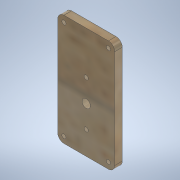
# Autodesk Inventor part: 上下直動t5.5_エンコーダ軸受け_CPY
Saved by Autodesk Inventor 2020.3 (Build 243373000, 373)
## iProperties
Created: 2020-07-07
Part Number: 上下直動t5.5_エンコーダ軸受け_CPY
Material: 木材 (カエデ材)
Document SubType Name: Modeling
Designer: totot
Density: 0.67 g/cm^3
Appearance: ナチュラル カエデ材 - 光沢 濃い着色
Author: totot
Autodesk Inventor part; units mm, degrees
ref_plane "YZ Plane" through (0, 0, 0) normal (1, 0, 0) x (0, 1, 0)
ref_plane "XZ Plane" through (0, 0, 0) normal (0, 1, 0) x (-1, 0, 0)
ref_plane "XY Plane" through (0, 0, 0) normal (0, 0, 1) x (1, 0, 0)
sketch "スケッチ1" plane through (0, 0, 0) normal (0, 0, 1) x (1, 0, 0)
  line L0 (0, 0) -> (41, 0)
  line L1 (41, 0) -> (41, -80)
  line L2 (41, -80) -> (0, -80)
  line L3 (0, -80) -> (0, 0)
  dimension "d0" = 41
  dimension "d13" = 80
  constraints: 8 end point, 2 parallel, 1 horizontal, 1 perpendicular
  measures "d0" distance of L1.end L2.end
  measures "d13" distance between parallel lines of L2 L0
extrude "押し出し1" add sketch "スケッチ1" along normal blind 5.5
sketch "スケッチ2" plane through (0, 0, 5.5) normal (0, 0, 1) x (1, 0, 0)
  line L0 (4.5, -75.5) -> (36.5, -75.5)
  line L1 (36.5, -75.5) -> (36.5, -4.5)
  line L2 (36.5, -4.5) -> (4.5, -4.5)
  line L3 (4.5, -4.5) -> (4.5, -75.5)
  line L4 (0, -80) -> (41, -80) projected
  line L5 (0, 0) -> (0, -80) projected
  dimension "d3" = 4.5
  dimension "d4" = 32
  dimension "d5" = 4.5
  dimension "d14" = 71
  constraints: 8 end point, 4 coincident, 2 parallel, 1 horizontal, 1 perpendicular
  measures "d3" distance between parallel lines of L4 L0
  measures "d4" distance of L1.end L2.end
  measures "d5" distance between parallel lines of L5 L3
  measures "d14" distance of L2.end L0.start
hole "穴1" at (4.5, -4.5, 5.5) at (36.5, -4.5, 5.5) at (36.5, -75.5, 5.5) at (4.5, -75.5, 5.5) direction (0, 0, -1) diameter 3 end through all
fillet "フィレット1" radius 4.5 4 edges at (0, 0, 2.75) (41, 0, 2.75) (0, -80, 2.75) (41, -80, 2.75)
sketch "スケッチ3" plane through (0, 0, 5.5) normal (0, 0, 1) x (1, 0, 0)
  line L0 (36.5, 0) -> (4.5, 0) projected
  line L1 (41, -75.5) -> (41, -4.5) projected
  line L2 (0, -4.5) -> (0, -75.5) projected
  point P0 (0, 0)
  point P1 (20.5, -47)
  dimension "d16" = 47
  dimension "d17" = 41
  dimension "d18" = 20.5
  measures "d16" distance from line of point (20.5, -47) L0
  measures "d17" distance between parallel lines of L1 L2
  measures "d18" distance from line of point (20.5, -47) L2
hole "穴2" at (20.5, -47, 5.5) direction (0, 0, -1) diameter 6 end through all
sketch "スケッチ4" plane through (0, 0, 5.5) normal (0, 0, 1) x (1, 0, 0)
  circle A0 centre (20.5, -47) radius 3 projected
  point P0 (0, 0)
  point P1 (20.5, -30.785)
  point P2 (20.5, -63.215)
  dimension "d26" = 32.43
  dimension "d27" = 16.215
  dimension "d28" = 0
  dimension "d29" = 0
  measures "d26" distance of point (20.5, -63.215) point (20.5, -30.785)
  measures "d27" distance of A0.centre point (20.5, -30.785)
  measures "d28" horizontal distance of point (20.5, -30.785) A0.centre
  measures "d29" horizontal distance of point (20.5, -63.215) A0.centre
hole "穴3" at (20.5, -30.785, 5.5) at (20.5, -63.215, 5.5) direction (0, 0, -1) diameter 3 end through all
equation "\"d18\" = 0.5 * d17"
equation "\"d27\" = 0.5 * d26"
